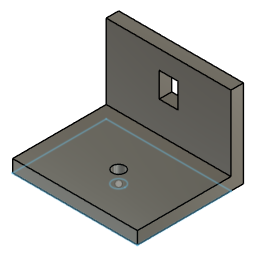
kat 2 v1 (Autodesk Fusion 360 design; units mm, degrees)
Autodesk Fusion 360 part; units mm, degrees
sketch "Szkic1" plane through (0, 0, 0) normal (0, 0, 1) x (1, 0, 0)
  line L0 (-10, 10) -> (10, 10)
  line L1 (10, 10) -> (10, -5)
  line L2 (10, -5) -> (-10, -5)
  line L3 (-10, -5) -> (-10, 10)
  circle A0 centre (0, 2) radius 1
  dimension "d1" = 15
  dimension "d10" = 2
  constraint horizontal L0
  constraint vertical L1
  constraint horizontal L2
  constraint vertical L3
  measures "d1" distance of L0.end L1.end
  measures "d10" diameter of A0
extrude "Wyciągnięcie proste1" add sketch "Szkic1" along normal blind 2 contours L0 L1 L2 L3 | A0
sketch "Szkic2" plane through (0, 10, 0) normal (0, 1, 0) x (-1, 0, 0)
  line L0 (-10, 0) -> (10, 0)
  line L1 (10, 0) -> (10, 2)
  line L2 (10, 2) -> (-10, 2)
  line L3 (-10, 2) -> (-10, 0)
  line L4 (-10, 0) -> (10, 0)
  line L5 (10, 0) -> (10, 14)
  line L6 (10, 14) -> (-10, 14)
  line L7 (-10, 14) -> (-10, 0)
  line L8 (1.5, 11) -> (-1.5, 11)
  line L9 (-1.5, 11) -> (-1.5, 7)
  line L10 (-1.5, 7) -> (1.5, 7)
  line L11 (1.5, 7) -> (1.5, 11)
  dimension "d4" = 8.5
  dimension "d5" = 3
  dimension "d6" = 20
  dimension "d7" = 3
  constraint horizontal L4
  constraint vertical L5
  constraint horizontal L6
  constraint vertical L7
  constraint coincident L0.start L3.end
  constraint horizontal L8
  constraint vertical L9
  constraint horizontal L10
  constraint vertical L11
  measures "d4" distance of L5 L11
  measures "d5" distance of L8.start L8.end
  measures "d6" distance of L5.end L6.end
  measures "d7" distance of L6 L8
extrude "Wyciągnięcie proste2" add sketch "Szkic2" along normal blind 2
extrude "Wyciągnięcie proste3" cut sketch "Szkic1" along normal blind 3 contours A0
